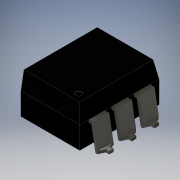
# Autodesk Inventor part: H11L1M
Saved by Autodesk Inventor 2016 (Build 200138000, 138)
## iProperties
Created: 2016-08-10
Part Number: H11L1M
Material: Generic
Document SubType Name: Modeling
Designer: jfixelle
Density: 1 g/cm^3
Appearance: Black
Author: jfixelle
Autodesk Inventor part; units mm, degrees
ref_plane "YZ Plane" through (0, 0, 0) normal (1, 0, 0) x (0, 1, 0)
ref_plane "XZ Plane" through (0, 0, 0) normal (0, 1, 0) x (-1, 0, 0)
ref_plane "XY Plane" through (0, 0, 0) normal (0, 0, 1) x (1, 0, 0)
sketch "Sketch1" plane through (0, 0, 0) normal (0, 1, 0) x (-1, 0, 0)
  line L0 (3.3, 4.445) -> (-3.3, 4.445)
  line L1 (-3.3, 4.445) -> (-3.3, -4.445)
  line L2 (-3.3, -4.445) -> (3.3, -4.445)
  line L3 (3.3, -4.445) -> (3.3, 4.445)
  point P0 (0, 0)
  dimension "d0" = 8.89
  dimension "d1" = 4.445
  dimension "d2" = 6.6
  dimension "d3" = 3.3
  constraints: 8 end point, 2 parallel, 1 horizontal, 1 perpendicular
  measures "d0" distance of L2.end L0.start
  measures "d1" distance from line of L2 point (0, 0)
  measures "d2" distance of L1.end L2.end
  measures "d3" distance from line of L3 point (0, 0)
extrude "Extrusion1" add sketch "Sketch1" along normal blind 4.38
chamfer "Chamfer1" distance 1.89 angle 10 1 edges at (3.3, 4.38, 0) measured on face at (3.3, 1.46, 1.4817)
chamfer "Chamfer2" distance 1.89 angle 10 1 edges at (-0.1666, 4.38, 4.445) measured on face at (-1.1, 2.29, 4.445)
chamfer "Chamfer3" distance 1.89 angle 10 1 edges at (-0.1666, 4.38, -4.445) measured on face at (-1.1, 2.29, -4.445)
sketch "Sketch2" plane through (0, 0, 0) normal (0, 0, 1) x (1, 0, 0)
  line L0 (3.3, 2.49) -> (3.3, 2.19)
  line L1 (3.3, 2.19) -> (3.5877, 2.19)
  line L2 (3.5877, 2.19) -> (4.065, -0.38)
  line L3 (4.065, -0.38) -> (4.945, -0.38)
  line L4 (4.945, -0.38) -> (4.945, -0.08)
  line L5 (4.945, -0.08) -> (4.259, -0.08)
  line L6 (4.259, -0.08) -> (3.8058, 2.49)
  line L7 (3.8058, 2.49) -> (3.3, 2.49)
  line L8 (3.3, 0) -> (3.3, 2.49) projected
  line L9 (3.3, 0) -> (-3.3, 0) projected
  point P0 (0, 0)
  dimension "d27" = 0.3
  dimension "d30" = 0.765
  dimension "d31" = 0.88
  dimension "d32" = 0.38
  dimension "d33" = 2.49
  dimension "d34" = 0.3
  dimension "d35" = 0
  dimension "d36" = 100
  constraints: 16 end point, 3 perpendicular, 2 vertical, 1 parallel
  measures "d27" distance of L3.end L4.end
  measures "d30" distance from line of L8 L2.end
  measures "d31" distance from line of L4 L2.end
  measures "d32" distance between parallel lines of L9 L3
  measures "d33" distance between parallel lines of L7 L9
  measures "d34" distance of L0.start L0.end
  measures "d35" distance between parallel lines of L8 L0
  measures "d36" angle of L6 L5
extrude "Extrusion2" add sketch "Sketch2" along normal mid plane 1.78
sketch "Sketch3" plane through (4.259, -0.08, 0.89) normal (0, 1, 0) x (1, 0, 0)
  line L0 (0.289, 1.14) -> (0.01, 1.78)
  line L1 (0.01, 1.78) -> (0.686, 1.78)
  line L2 (0.686, 1.78) -> (0.686, 1.14)
  line L3 (0.686, 1.78) -> (0.686, 0) projected
  line L4 (0.686, 1.14) -> (0.289, 1.14)
  line L5 (0.686, 1.78) -> (0.686, 0) projected
  point P0 (-4.259, 0.89)
  dimension "d41" = 0.64
  constraints: 8 end point, 2 perpendicular
  measures "d41" distance between parallel lines of L1 L4
extrude "Extrusion3" cut sketch "Sketch3" against normal up to next
mirror "Mirror1" about plane through (0, 0, 0) normal (0, 0, 1) of "Extrusion3"
pattern_linear "Rectangular Pattern1" count 3 spacing 2.54 along (0, 0, 1) of "Extrusion2", "Extrusion3", "Mirror1" first direction both ways yes
mirror "Mirror2" about plane through (0, 0, 0) normal (1, 0, 0) of "Extrusion2", "Extrusion3", "Mirror1", "Rectangular Pattern1"
sketch "Sketch4" plane through (0, 4.38, 0) normal (0, 1, 0) x (1, 0, 0)
  circle A0 centre (2.0844, -3.3612) radius 0.3556
  point P0 (0, 0)
  constraints: 1 centre point
extrude "Extrusion4" cut sketch "Sketch4" against normal blind 0.05
body "Solid1"
